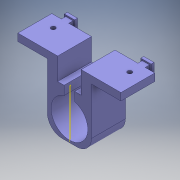
# Autodesk Inventor part: support_codeur
Saved by Autodesk Inventor 2019 (Build 230136000, 136)
## iProperties
Created: 2017-12-27
Part Number: support_codeur
Material: Generic
Document SubType Name: Modeling
Designer: franc
Density: 1 g/cm^3
Appearance: Default
Mass: 18.7729 g
Surface Area: 102.906 cm^2
Volume: 18.7729 cm^3
Author: franc
Autodesk Inventor part; units mm, degrees
ref_plane "YZ Plane" through (0, 0, 0) normal (1, 0, 0) x (0, 1, 0)
ref_plane "XZ Plane" through (0, 0, 0) normal (0, 1, 0) x (-1, 0, 0)
ref_plane "XY Plane" through (0, 0, 0) normal (0, 0, 1) x (1, 0, 0)
sketch "Esquisse1" plane through (0, 0, 0) normal (0, 1, 0) x (-1, 0, 0)
  line L0 (7.2872, 10.2128) -> (-22.7128, 10.2128)
  line L1 (-22.7128, 10.2128) -> (-22.7128, -19.7872)
  line L2 (-22.7128, -19.7872) -> (7.2872, -19.7872)
  line L3 (7.2872, -19.7872) -> (7.2872, 10.2128)
  point P0 (0, 0)
  dimension "d0" = 30
  dimension "d1" = 30
  constraints: 8 end point, 2 parallel, 1 horizontal, 1 perpendicular
  measures "d0" distance of L2.end L0.start
  measures "d1" distance of L0.start L0.end
extrude "Extrusion1" add sketch "Esquisse1" along normal blind 23
ref_plane "Plan médian" through (7.7128, 0, 10.2128) normal (1, 0, 0) x (0, 0, -1)
sketch "Esquisse4" plane through (0, 0, 0) normal (0, -1, 0) x (1, 0, 0)
  circle A0 centre (7.7128, -7.8122) radius 11.975 projected
  line L0 (-7.2872, 10.2128) -> (22.7128, 10.2128) projected
  line L1 (4.1002, 3.6049) -> (4.1002, 10.2128)
  line L2 (11.3254, 3.6049) -> (11.3254, 10.2128)
  point P0 (0, 0)
  constraints: 4 end point, 2 point on circle, 2 point on line, 2 vertical, 1 other
extrude "Extrusion2" cut sketch "Esquisse4" against normal blind 22
sketch "Esquisse5" plane through (0, 22, 0) normal (0, -1, 0) x (1, 0, 0)
  circle A0 centre (15.507, -3.3122) radius 1.25 projected
  circle A1 centre (-0.0815, -3.3122) radius 1.25 projected
  circle A2 centre (7.7128, -16.8122) radius 1.25 projected
  circle A3 centre (7.7128, -7.8122) radius 6 projected
  point P0 (0, 0)
extrude "Extrusion3" cut sketch "Esquisse5" against normal through all
sketch "Esquisse6" plane through (-7.2872, 23, 10.2128) normal (0, 0, 1) x (1, 0, 0)
  line L0 (0, -23) -> (11.3874, -23) projected
  line L1 (5.9558, 0) -> (8.4558, 0) projected
  line L2 (0, -23) -> (7, -23)
  line L3 (7, -23) -> (7, 0)
  line L4 (7, 0) -> (0, 0)
  line L5 (0, 0) -> (0, -23)
  line L6 (30, -23) -> (30, 0) projected
  line L7 (0, 0) -> (30, 0) projected
  line L8 (30, -23) -> (23, -23)
  line L9 (23, -23) -> (23, 0)
  line L10 (23, 0) -> (30, 0)
  line L11 (30, 0) -> (30, -23)
  point P0 (7.2872, -23)
  point P1 (12, -23)
  point P2 (11.5355, -23)
  dimension "d8" = 7
  dimension "d9" = 7
  constraints: 16 end point, 4 parallel, 2 horizontal, 2 perpendicular, 2 point on line
  measures "d8" distance between parallel lines of L5 L3
  measures "d9" distance between parallel lines of L6 L9
extrude "Extrusion4" add sketch "Esquisse6" along normal blind 10
sketch "Esquisse7" plane through (-7.2872, 23, 20.2128) normal (0, 0, 1) x (1, 0, 0)
  line L0 (7, 0) -> (-20, 0)
  line L1 (-20, 0) -> (-20, -23)
  line L2 (-20, -23) -> (7, -23)
  line L3 (7, -23) -> (7, 0)
  line L4 (30, 0) -> (0, 0) projected
  line L5 (23, 0) -> (50, 0)
  line L6 (50, 0) -> (50, -23)
  line L7 (50, -23) -> (23, -23)
  line L8 (23, -23) -> (23, 0)
  line L9 (0, 0) -> (0, -23) projected
  line L10 (30, -23) -> (30, 0) projected
  point P0 (7.2872, -23)
  dimension "d12" = 20
  dimension "d13" = 20
  constraints: 16 end point, 4 parallel, 2 horizontal, 2 perpendicular, 1 point on line
  measures "d12" distance between parallel lines of L1 L9
  measures "d13" distance between parallel lines of L6 L10
extrude "Extrusion5" add sketch "Esquisse7" along normal blind 5
sketch "Esquisse8" plane through (0, 23, 0) normal (0, 1, 0) x (1, 0, 0)
  line L0 (36.2128, -25.2128) -> (31.2128, -25.2128)
  line L1 (31.2128, -25.2128) -> (31.2128, -20.2128)
  line L2 (31.2128, -20.2128) -> (36.2128, -20.2128)
  line L3 (36.2128, -20.2128) -> (36.2128, -25.2128)
  line L4 (42.7128, -20.2128) -> (42.7128, -25.2128) projected
  line L5 (42.7128, -20.2128) -> (22.7128, -20.2128) projected
  line L6 (-0.2872, -25.2128) -> (-27.2872, -25.2128) projected
  line L7 (-27.2872, -20.2128) -> (-27.2872, -25.2128) projected
  line L8 (-20.7872, -25.2128) -> (-15.7872, -25.2128)
  line L9 (-15.7872, -25.2128) -> (-15.7872, -20.2128)
  line L10 (-15.7872, -20.2128) -> (-20.7872, -20.2128)
  line L11 (-20.7872, -20.2128) -> (-20.7872, -25.2128)
  line L12 (-7.2872, -20.2128) -> (-27.2872, -20.2128) projected
  point P0 (0, 0)
  point P1 (-0.4939, -25.2128)
  dimension "d16" = 6.5
  dimension "d17" = 5
  dimension "d18" = 5
  dimension "d19" = 0
  dimension "d53" = 5
  dimension "d54" = 5
  dimension "d55" = 0
  dimension "d57" = 6.5
  constraints: 16 end point, 4 parallel, 2 horizontal, 2 perpendicular
  measures "d16" distance between parallel lines of L4 L3
  measures "d17" distance of L2.end L0.start
  measures "d18" distance of L0.start L0.end
  measures "d19" distance between parallel lines of L5 L2
  measures "d53" distance of L10.end L9.end
  measures "d54" distance of L10.end L8.start
  measures "d55" distance between parallel lines of L12 L10
  measures "d57" distance between parallel lines of L7 L11
extrude "Extrusion6" add sketch "Esquisse8" along normal blind 3 contours L0 L1 L2 L3 | L6 L11 L10 L9
sketch "Esquisse9" plane through (0, 26, 0) normal (0, 1, 0) x (1, 0, 0)
  line L0 (37.2128, -26.2128) -> (30.2128, -26.2128)
  line L1 (30.2128, -26.2128) -> (30.2128, -19.2128)
  line L2 (30.2128, -19.2128) -> (37.2128, -19.2128)
  line L3 (37.2128, -19.2128) -> (37.2128, -26.2128)
  line L4 (42.7128, -20.2128) -> (42.7128, -25.2128) projected
  line L5 (-27.2872, -25.2128) -> (-0.2872, -25.2128) projected
  line L6 (-27.2872, -20.2128) -> (-27.2872, -25.2128) projected
  line L7 (31.2128, -25.2128) -> (15.7128, -25.2128) projected
  line L8 (-14.7872, -26.2128) -> (-21.7872, -26.2128)
  line L9 (-21.7872, -26.2128) -> (-21.7872, -19.2128)
  line L10 (-21.7872, -19.2128) -> (-14.7872, -19.2128)
  line L11 (-14.7872, -19.2128) -> (-14.7872, -26.2128)
  point P0 (0, 0)
  point P1 (-13.7872, -25.2128)
  dimension "d25" = 7
  dimension "d26" = 5.5
  dimension "d59" = 7
  dimension "d60" = 1
  dimension "d62" = 5.5
  dimension "d63" = 1
  dimension "d64" = 7
  dimension "d65" = 7
  constraints: 16 end point, 4 parallel, 2 horizontal, 2 perpendicular, 1 midpoint
  measures "d25" distance between parallel lines of L1 L3
  measures "d26" distance between parallel lines of L4 L3
  measures "d59" distance between parallel lines of L2 L0
  measures "d60" distance between parallel lines of L7 L0
  measures "d62" distance between parallel lines of L6 L9
  measures "d63" distance between parallel lines of L5 L8
  measures "d64" distance of L8.end L9.end
  measures "d65" distance of L9.end L10.end
extrude "Extrusion7" add sketch "Esquisse9" along normal blind 2
sketch "Esquisse10" plane through (22.7128, 23, -19.7872) normal (0, 0, -1) x (-1, 0, 0)
  line L0 (0, -23) -> (15, -23) projected
  line L1 (15, -23) -> (15, -1) projected
  line L2 (15, -23) -> (30, -23) projected
  line L3 (30, -23) -> (30, 0) projected
  line L4 (0, 0) -> (30, 0) projected
  line L5 (0, -23) -> (0, 0) projected
  line L6 (0, 0) -> (30, 0)
  line L7 (30, 0) -> (30, -23)
  line L8 (30, -23) -> (0, -23)
  line L9 (0, -23) -> (0, 0)
  point P0 (22.7128, -23)
  constraints: 8 end point, 2 parallel, 1 horizontal, 1 perpendicular
extrude "Extrusion8" add sketch "Esquisse10" along normal blind 2
fillet "Congé1" radius 10 2 edges at (22.7128, 11.5, -21.7872) (-7.2872, 11.5, -21.7872)
sketch "Esquisse12" plane through (0, 0, 0) normal (0, -1, 0) x (1, 0, 0)
  arc A0 (4.1002, 3.6049) -> (11.3254, 3.6049) centre (7.7128, -7.8122) ccw projected
  circle A1 centre (7.7128, -7.8122) radius 12.5
  point P0 (0, 0)
  dimension "d42" = 25
  constraints: 1 centre point, 1 coincident
  measures "d42" diameter of A1
extrude "Extrusion10" cut sketch "Esquisse12" against normal up to surface (22 mm away)
sketch "Esquisse13" plane through (-7.2872, 23, 25.2128) normal (0, 0, 1) x (1, 0, 0)
  circle A0 centre (-11, -8) radius 1.5
  circle A1 centre (41, -8) radius 1.5
  line L0 (7, 0) -> (-20, 0) projected
  line L1 (-20, 0) -> (-20, -23) projected
  line L2 (50, 0) -> (23, 0) projected
  line L3 (50, -23) -> (50, 0) projected
  point P0 (7.2872, -23)
  dimension "d45" = 3
  dimension "d46" = 3
  dimension "d49" = 8
  dimension "d50" = 9
  dimension "d51" = 8
  dimension "d52" = 9
  constraints: 2 centre point
  measures "d45" diameter of A0
  measures "d46" diameter of A1
  measures "d49" distance from line of L0 A0.centre
  measures "d50" distance from line of L1 A0.centre
  measures "d51" distance from line of L2 A1.centre
  measures "d52" distance from line of L3 A1.centre
extrude "Extrusion11" cut sketch "Esquisse13" against normal through all
